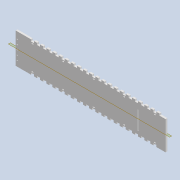
# Autodesk Inventor part: 10_Baseplate_Simmo_side1
Saved by Autodesk Inventor 2022 (Build 260153000, 153)
## iProperties
Created: 2022-08-04
Part Number: 10_Baseplate_Simmo_side1
Material: Generic
Document SubType Name: Modeling
Designer: wanghaoran
Density: 1 g/cm^3
Appearance: Default
Author: wanghaoran
Autodesk Inventor part; units mm, degrees
ref_plane "YZ Plane" through (0, 0, 0) normal (1, 0, 0) x (0, 1, 0)
ref_plane "XZ Plane" through (0, 0, 0) normal (0, 1, 0) x (-1, 0, 0)
ref_plane "XY Plane" through (0, 0, 0) normal (0, 0, 1) x (1, 0, 0)
sketch "Sketch1" plane through (0, 0, 0) normal (0, 0, 1) x (1, 0, 0)
  line L0 (4.9654, 0) -> (4.9654, 6) projected
  line L1 (-450, -9) -> (-450, -67) projected
  line L2 (40, 0) -> (40, 6) projected
  line L3 (40, 6) -> (-450, 6)
  line L4 (-450, 6) -> (-450, -94)
  line L5 (-450, -94) -> (40, -94)
  line L6 (40, -94) -> (40, 6)
  point P0 (-450, -9)
  point P1 (-450, -67)
  dimension "d26" = 490
  dimension "d27" = 100
  constraints: 8 end point, 2 parallel, 1 horizontal, 1 perpendicular
  measures "d26" distance of L5.end L4.end
  measures "d27" distance of L4.end L3.end
extrude "Extrusion1" add sketch "Sketch1" along normal blind 6
sketch "Sketch2" plane through (0, 0, 6) normal (0, 0, 1) x (1, 0, 0)
  line L0 (-10, 0) -> (-10, 6) projected
  line L1 (-20, 6) -> (-10, 6) projected
  line L2 (-20, 6) -> (-20, 0) projected
  line L3 (-20, 0) -> (-10, 0) projected
  line L4 (-10, 6) -> (-9.9, 6)
  line L5 (-9.9, 6) -> (-9.9, 0)
  line L6 (-9.9, 0) -> (-10, 0)
  line L7 (-10, 0) -> (-10, 6)
  line L8 (-20, 6) -> (-20.1, 6)
  line L9 (-20.1, 6) -> (-20.1, 0)
  line L10 (-20.1, 0) -> (-20, 0)
  line L11 (-20, 0) -> (-20, 6)
  point P0 (0, 0)
  dimension "d5" = 0.1
  dimension "d6" = 0.1
  constraints: 16 end point, 4 parallel, 2 horizontal, 2 perpendicular, 1 point on line
  measures "d5" distance of L5.end L6.end
  measures "d6" distance of L10.end L9.end
extrude "Extrusion2" cut sketch "Sketch2" against normal blind 6
pattern_linear "Rectangular Pattern1" count 20 spacing 20 along (-1, 0, 0) of "Extrusion2"
ref_plane "Work Plane1" through (-450, -44, 0) normal (0, -1, 0) x (1, 0, 0)
sketch "Sketch4" plane through (0, 0, 6) normal (0, 0, 1) x (1, 0, 0)
  circle A0 centre (-445, -76.5) radius 1.6
  line L0 (-445, -76.5) -> (-445, -54)
  circle A1 centre (-445, -61.5) radius 1.6
  circle A2 centre (-445, -46.5) radius 1.6
  circle A3 centre (-445, -31.5) radius 1.6
  circle A4 centre (-445, -16.5) radius 1.6
  line L1 (-450, -94) -> (40, -94) projected
  line L2 (-450, 6) -> (-450, -94) projected
  point P0 (0, 0)
  dimension "d15" = 3.2
  dimension "d18" = 15
  dimension "d46" = 17.5
  dimension "d47" = 5
  constraints: 5 centre point, 2 end point, 1 vertical, 8 other
  measures "d15" diameter of A0
  measures "d18" distance of L0.start A1.centre
  measures "d46" distance from line of L1 L0.start
  measures "d47" distance from line of L2 L0.start
extrude "Extrusion4" cut sketch "Sketch4" against normal blind 6
pattern_linear "Rectangular Pattern3" count 2 spacing 20 along (1, 0, 0) of "Extrusion2"
sketch "Sketch5" plane through (0, 0, 6) normal (0, 0, 1) x (1, 0, 0)
  line L0 (20, 0) -> (40, 0) projected
  line L1 (20, 6) -> (20, 0) projected
  line L2 (20, 6) -> (40, 6) projected
  line L3 (40, 0) -> (40, 6) projected
  point P0 (0, 0)
extrude "Extrusion5" cut sketch "Sketch5" against normal through all
mirror "Mirror3" about plane through (-450, -44, 0) normal (0, -1, 0) of "Extrusion2", "Rectangular Pattern1"
mirror "Mirror4" about plane through (-450, -44, 0) normal (0, -1, 0) of "Extrusion2", "Rectangular Pattern3"
sketch "Sketch6" plane through (0, 0, 6) normal (0, 0, 1) x (1, 0, 0)
  line L0 (7.75, -5.4) -> (2.25, -5.4)
  line L1 (2.25, -5.4) -> (2.25, -3)
  line L2 (2.25, -3) -> (7.75, -3)
  line L3 (7.75, -3) -> (7.75, -5.4)
  line L4 (-0.1, 0) -> (-0.1, 6) projected
  line L5 (10.1, 0) -> (-0.1, 0) projected
  line L6 (-97.75, -3) -> (-92.25, -3)
  line L7 (-92.25, -5.4) -> (-97.75, -5.4)
  line L8 (-97.75, -5.4) -> (-97.75, -3)
  line L9 (-92.25, -3) -> (-92.25, -5.4)
  line L10 (-197.75, -3) -> (-192.25, -3)
  line L11 (-192.25, -5.4) -> (-197.75, -5.4)
  line L12 (-197.75, -5.4) -> (-197.75, -3)
  line L13 (-192.25, -3) -> (-192.25, -5.4)
  line L14 (-297.75, -3) -> (-292.25, -3)
  line L15 (-292.25, -5.4) -> (-297.75, -5.4)
  line L16 (-297.75, -5.4) -> (-297.75, -3)
  line L17 (-292.25, -3) -> (-292.25, -5.4)
  line L18 (-397.75, -3) -> (-392.25, -3)
  line L19 (-392.25, -5.4) -> (-397.75, -5.4)
  line L20 (-397.75, -5.4) -> (-397.75, -3)
  line L21 (-392.25, -3) -> (-392.25, -5.4)
  point P0 (0, 0)
  dimension "d33" = 5.5
  dimension "d34" = 2.4
  dimension "d35" = 2.35
  dimension "d36" = 3
  dimension "d39" = 100
  constraints: 40 end point, 2 horizontal, 2 parallel, 1 perpendicular, 32 other
  measures "d33" distance of L1.end L2.end
  measures "d34" distance of L0.end L1.end
  measures "d35" distance between parallel lines of L4 L1
  measures "d36" distance between parallel lines of L5 L2
  measures "d39" distance of L1.end L6.start
extrude "Extrusion6" cut sketch "Sketch6" against normal through all
mirror "Mirror5" about plane through (-450, -44, 0) normal (0, -1, 0) of "Extrusion6"
sketch "Sketch7" plane through (0, 0, 6) normal (0, 0, 1) x (1, 0, 0)
  line L0 (-44.2445, -65.933) -> (-44.2445, -17.933) projected
  line L1 (-46.2142, -65.933) -> (-44.2445, -65.933) projected
  line L2 (-46.2142, -65.933) -> (-46.2142, -17.933) projected
  line L3 (-46.2142, -17.933) -> (-44.2445, -17.933) projected
  line L4 (-49.2142, -17.933) -> (-51.2142, -17.933)
  line L5 (-51.2142, -17.933) -> (-51.2142, -77.933)
  line L6 (-51.2142, -77.933) -> (-49.2142, -77.933)
  line L7 (-49.2142, -77.933) -> (-49.2142, -17.933)
  point P0 (0, 0)
  point P1 (-46.2142, -12.933)
  dimension "d61" = 2
  dimension "d62" = 60
  dimension "d63" = 3
  constraints: 8 end point, 2 parallel, 1 horizontal, 1 perpendicular
  measures "d61" distance of L6.end L5.end
  measures "d62" distance of L5.end L4.end
  measures "d63" distance between parallel lines of L7 L2
extrude "Extrusion7" cut sketch "Sketch7" against normal through all contours L7 L6 L5 L4
body "Solid1"
